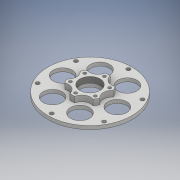
# Autodesk Inventor part: PortaCoronasCassette
Saved by Autodesk Inventor 2018 (Build 220112000, 112)
## iProperties
Created: 2017-05-06
Part Number: PortaCoronasCassette
Material: Generic
Document SubType Name: Modeling
Designer: eroldan
Density: 1 g/cm^3
Appearance: Default
Author: eroldan
Autodesk Inventor part; units mm, degrees
ref_plane "YZ Plane" through (0, 0, 0) normal (1, 0, 0) x (0, 1, 0)
ref_plane "XZ Plane" through (0, 0, 0) normal (0, 1, 0) x (-1, 0, 0)
ref_plane "XY Plane" through (0, 0, 0) normal (0, 0, 1) x (1, 0, 0)
sketch "Sketch1" plane through (0, 0, 0) normal (0, 0, 1) x (1, 0, 0)
  circle A0 centre (0, 0) radius 17.5
  circle A1 centre (-47.5262, 0) radius 16.5
  circle A2 centre (0, 0) radius 73
  circle A3 centre (-23.7631, -41.1589) radius 16.5
  circle A4 centre (23.7631, -41.1589) radius 16.5
  circle A5 centre (47.5262, 0) radius 16.5
  circle A6 centre (23.7631, 41.1589) radius 16.5
  circle A7 centre (-23.7631, 41.1589) radius 16.5
  point P0 (0, 66.675)
  point P1 (-57.7422, 33.3375)
  point P2 (-57.7422, -33.3375)
  point P3 (0, -66.675)
  point P4 (57.7422, -33.3375)
  point P5 (57.7422, 33.3375)
  point P6 (0, 25)
  point P7 (-21.6506, 12.5)
  point P8 (-21.6506, -12.5)
  point P9 (0, -25)
  point P10 (21.6506, -12.5)
  point P11 (21.6506, 12.5)
  dimension "d0" = 66.675
  dimension "d3" = 360
  dimension "d9" = 35
  dimension "d19" = 33
  dimension "d20" = 25
  dimension "d23" = 360
  dimension "d25" = 146
  dimension "d28" = 360
  constraints: 8 centre point, 1 coincident, 27 other
  measures "d0" distance of point (0, 0) point (0, 66.675)
  measures "d9" diameter of A0
  measures "d19" diameter of A1
  measures "d20" distance of point (0, 25) point (0, 0)
  measures "d25" diameter of A2
extrude "Extrusion2" add sketch "Sketch1" along normal blind 6
hole "Hole2" at (0, 66.675, 0) at (-57.7422, 33.3375, 0) at (-57.7422, -33.3375, 0) at (0, -66.675, 0) at (57.7422, -33.3375, 0) at (57.7422, 33.3375, 0) direction (0, 0, 1) diameter 6.5 end through all
hole "Hole3" at (0, 25, 0) at (-21.6506, 12.5, 0) at (-21.6506, -12.5, 0) at (0, -25, 0) at (21.6506, 12.5, 0) at (21.6506, -12.5, 0) direction (0, 0, 1) diameter 5 end through all
sketch "Sketch3" plane through (0, 0, 6) normal (0, 0, 1) x (1, 0, 0)
  circle A0 centre (0, 0) radius 17.5 projected
  circle A1 centre (21.6506, 12.5) radius 2.5 projected
  circle A2 centre (0, 25) radius 2.5 projected
  circle A3 centre (-21.6506, 12.5) radius 2.5 projected
  circle A4 centre (-21.6506, -12.5) radius 2.5 projected
  circle A5 centre (0, -25) radius 2.5 projected
  circle A6 centre (21.6506, -12.5) radius 2.5 projected
  line L0 (0, 0) -> (23.058, 39.9377) construction
  line L1 (0, 0) -> (46.116, 0) construction
  arc A7 (4.3567, 30.6923) -> (24.402, 19.1191) centre (19.1506, 33.1699) ccw
  arc A8 (-24.402, 19.1191) -> (-4.3567, 30.6923) centre (-19.1506, 33.1699) ccw
  arc A9 (-28.7587, -11.5732) -> (-28.7587, 11.5732) centre (-38.3013, 0) ccw
  arc A10 (-4.3567, -30.6923) -> (-24.402, -19.1191) centre (-19.1506, -33.1699) ccw
  arc A11 (24.402, -19.1191) -> (4.3567, -30.6923) centre (19.1506, -33.1699) ccw
  arc A12 (28.7587, 11.5732) -> (28.7587, -11.5732) centre (38.3013, 0) ccw
  arc A13 (4.3567, 30.6923) -> (-4.3567, 30.6923) centre (0, 0) ccw
  arc A14 (-24.402, 19.1191) -> (-28.7587, 11.5732) centre (0, 0) ccw
  arc A15 (-28.7587, -11.5732) -> (-24.402, -19.1191) centre (0, 0) ccw
  arc A16 (-4.3567, -30.6923) -> (4.3567, -30.6923) centre (0, 0) ccw
  arc A17 (24.402, -19.1191) -> (28.7587, -11.5732) centre (0, 0) ccw
  arc A18 (28.7587, 11.5732) -> (24.402, 19.1191) centre (0, 0) ccw
  dimension "d48" = 60
  dimension "d49" = 30
  dimension "d52" = 360
  constraints: 24 point on circle, 12 centre point, 4 end point, 1 coincident, 1 equal length, 1 horizontal, 1 point on line, 25 other
  measures "d48" angle of L1 L0
  measures "d49" diameter of A7
extrude "Extrusion3" add sketch "Sketch3" along normal blind 10 separate body
thread "Thread1" size "Rc 1/16" standard "DIN Pipe Taper Internal" length 10
